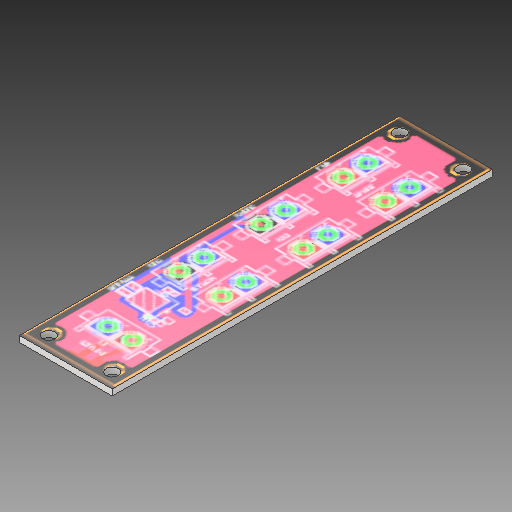
# Autodesk Inventor part: powerDist
Saved by Autodesk Inventor 2018 (Build 220112000, 112)
## iProperties
Created: 2018-08-04
Part Number: powerDist
Material: ABS Plastic
Document SubType Name: Modeling
Designer: Cole Tucker
Density: 1.06 g/cm^3
Appearance: Smooth - White
Mass: 4.00077 g
Surface Area: 51.754 cm^2
Volume: 3.77431 cm^3
Author: Cole Tucker
Autodesk Inventor part; units mm, degrees
ref_plane "YZ Plane" through (0, 0, 0) normal (1, 0, 0) x (0, 1, 0)
ref_plane "XZ Plane" through (0, 0, 0) normal (0, 1, 0) x (-1, 0, 0)
ref_plane "XY Plane" through (0, 0, 0) normal (0, 0, 1) x (1, 0, 0)
sketch "Sketch1" plane through (0, 0, 0) normal (0, 1, 0) x (-1, 0, 0)
  line L0 (0, 0) -> (24.13, 0)
  line L1 (24.13, 0) -> (24.13, -99.06)
  line L2 (24.13, -99.06) -> (0, -99.06)
  line L3 (0, -99.06) -> (0, 0)
  dimension "d0" = 24.13
  dimension "d1" = 99.06
  constraints: 8 end point, 2 parallel, 1 horizontal, 1 perpendicular
  measures "d0" distance of L1.end L2.end
  measures "d1" distance of L0.end L1.end
extrude "Extrusion1" add sketch "Sketch1" along normal blind 1.6002
sketch "Sketch2" plane through (0, 1.6002, 0) normal (0, 1, 0) x (1, 0, 0)
  line L0 (0, 0) -> (0, 99.06) construction
  line L1 (0, 0) -> (-20.32, 0) construction
  line L2 (-20.32, 0) -> (-20.32, 95.25) construction
  line L3 (-20.32, 95.25) -> (0, 95.25) construction
  line L4 (0, 95.25) -> (0, 0) construction
  line L5 (0, 95.25) -> (-3.81, 95.25) construction
  line L6 (0, 0) -> (-3.81, 0) construction
  line L7 (-3.81, 0) -> (-3.81, 3.81) construction
  line L8 (-3.81, 3.81) -> (0, 3.81) construction
  line L9 (0, 3.81) -> (0, 0) construction
  line L10 (-3.81, 3.81) -> (-20.32, 3.81) construction
  dimension "d4" = 20.32
  dimension "d5" = 95.25
  dimension "d6" = 3.81
  dimension "d7" = 3.81
  dimension "d8" = 3.81
  constraints: 20 end point, 4 coincident, 4 parallel, 3 perpendicular, 2 horizontal, 2 point on line
  measures "d4" distance of L2.end L3.end
  measures "d5" distance of L1.end L2.end
  measures "d6" distance of L3.end L5.end
  measures "d7" distance of L7.end L8.end
  measures "d8" distance of L6.end L7.end
hole "Hole1" at (-20.32, 1.6002, -3.81) at (-3.81, 1.6002, -3.81) at (-3.81, 1.6002, -95.25) at (-20.32, 1.6002, -95.25) direction (0, -1, 0) diameter 3.175 depth 25.4 tip angle 118
sketch "Sketch4" plane through (0, 1.6002, 0) normal (0, 1, 0) x (1, 0, 0)
  line L0 (-24.13, 0) -> (0, 0) projected
  line L1 (0, 99.06) -> (-24.13, 99.06) projected
  line L2 (-24.13, 0) -> (0, 0)
  line L3 (0, 0) -> (0, 99.06)
  line L4 (0, 99.06) -> (-24.13, 99.06)
  line L5 (-24.13, 99.06) -> (-24.13, 0)
  line L6 (-36.8322, -5.5807) -> (-36.8322, 103.313) construction
  line L7 (-36.8322, 103.313) -> (12.7861, 103.313) construction
  line L8 (12.7861, 103.313) -> (12.7861, -5.5807) construction
  line L9 (12.7861, -5.5807) -> (-36.8322, -5.5807) construction
  constraints: 8 end point, 2 parallel, 1 horizontal, 1 perpendicular, 2 other
decal "Decal1"
body "Solid1"
